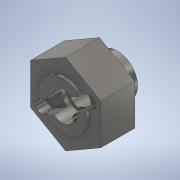
# Autodesk Inventor part: RCT-H009_tuerca
Saved by Autodesk Inventor 2020 (Build 240168000, 168)
## iProperties
Created: 2019-01-30
Part Number: RCT-H009_tuerca
Material: Generic
Document SubType Name: Modeling
Designer: Ehecatl Eli
Density: 1 g/cm^3
Appearance: Semi-Polished
Author: Ehecatl Eli
Autodesk Inventor part; units mm, degrees
ref_plane "YZ Plane" through (0, 0, 0) normal (1, 0, 0) x (0, 1, 0)
ref_plane "XZ Plane" through (0, 0, 0) normal (0, 1, 0) x (-1, 0, 0)
ref_plane "XY Plane" through (0, 0, 0) normal (0, 0, 1) x (1, 0, 0)
sketch "Sketch1" plane through (0, 0, 0) normal (0, 1, 0) x (-1, 0, 0)
  line L0 (0, -6.8127) -> (-5.9, -3.4064)
  line L1 (-5.9, -3.4064) -> (-5.9, 3.4064)
  line L2 (-5.9, 3.4064) -> (0, 6.8127)
  line L3 (0, 6.8127) -> (5.9, 3.4064)
  line L4 (5.9, 3.4064) -> (5.9, -3.4064)
  line L5 (5.9, -3.4064) -> (0, -6.8127)
  line L6 (0, -9.5378) -> (0, 9.5378) projected
  point P0 (0, 0)
  point P1 (0, 0)
  dimension "d0" = 11.8
  constraints: 12 end point, 1 coincident, 1 parallel, 13 other
  measures "d0" distance between parallel lines of L1 L4
extrude "Extrusion1" add sketch "Sketch1" along normal blind 5.7
sketch "Sketch2" plane through (0, 5.7, 0) normal (0, 1, 0) x (1, 0, 0)
  circle A0 centre (0, 0) radius 4.4
  dimension "d3" = 8.8
  constraints: 1 centre point, 1 coincident
  measures "d3" diameter of A0
extrude "Extrusion2" add sketch "Sketch2" along normal blind 1
sketch "Sketch3" plane through (0, 6.7, 0) normal (0, 1, 0) x (1, 0, 0)
  circle A0 centre (0, 0) radius 3.4
  dimension "d6" = 6.8
  constraints: 1 centre point, 1 coincident
  measures "d6" diameter of A0
extrude "Extrusion3" add sketch "Sketch3" along normal blind 2
sketch "Sketch4" plane through (0, 0, 0) normal (0, 1, 0) x (-1, 0, 0)
  circle A0 centre (0, 0) radius 4
  dimension "d9" = 8
  constraints: 1 centre point, 1 coincident
  measures "d9" diameter of A0
extrude "Extrusion4" add sketch "Sketch4" against normal blind 0.5
sketch "Sketch5" plane through (0, -0.5, 0) normal (0, -1, 0) x (1, 0, 0)
  circle A0 centre (0, 0) radius 2.5
  dimension "d12" = 5
  constraints: 1 centre point, 1 coincident
  measures "d12" diameter of A0
extrude "Extrusion5" cut sketch "Sketch5" against normal blind 3
sketch "Sketch6" plane through (0, 8.7, 0) normal (0, 1, 0) x (1, 0, 0)
  circle A0 centre (0, 0) radius 2
  dimension "d15" = 4
  constraints: 1 centre point, 1 coincident
  measures "d15" diameter of A0
extrude "Extrusion6" cut sketch "Sketch6" against normal up to next
sketch "Sketch7" plane through (0, -0.5, 0) normal (0, -1, 0) x (1, 0, 0)
  line L0 (-4.1136, -2.375) -> (4.1136, 2.375) construction
  line L1 (-3.6136, -3.241) -> (4.6136, 1.509)
  line L2 (3.6136, 3.241) -> (-4.6136, -1.509)
  arc A0 (-4.6136, -1.509) -> (-3.6136, -3.241) centre (-4.1136, -2.375) ccw
  arc A1 (4.6136, 1.509) -> (3.6136, 3.241) centre (4.1136, 2.375) ccw
  line L3 (0, 6.8127) -> (-5.9, 3.4064) projected
  point P0 (0, 0)
  point P1 (0, 0)
  dimension "d18" = 11.5
  dimension "d19" = 2
  constraints: 8 end point, 4 point on circle, 4 tangent, 2 centre point, 2 parallel, 1 coincident, 1 midpoint
  measures "d19" distance between parallel lines of L1 L2
extrude "Extrusion7" cut sketch "Sketch7" against normal blind 2.3
sketch "Sketch8" plane through (0, 0, -6.8127) normal (0.5, 0, -0.8660254) x (-0.8660254, 0, -0.5)
  line L0 (0, 0) -> (0, 5.7) construction
  line L1 (-6.8127, 0) -> (-6.8127, 5.7) construction
  circle A0 centre (-3.4064, 2) radius 1.5
  line L2 (9.6112, 0) -> (-21.9003, 0) projected
  point P0 (-3.4064, 0)
  dimension "d23" = 3
  dimension "d24" = 2
  dimension "d25" = 0
  constraints: 1 centre point
  measures "d23" diameter of A0
  measures "d24" distance from line of L2 A0.centre
  measures "d25" horizontal distance of A0.centre point (-3.406, 0)
extrude "Extrusion8" cut sketch "Sketch8" against normal up to surface
thread "Thread1" size "M3x0.5" class "6H" standard "ANSI Metric M Profile" full length
body "Solid1"
